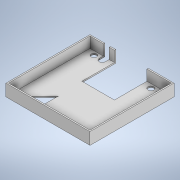
# Autodesk Inventor part: FixedLid
Saved by Autodesk Inventor 2020 (Build 240168000, 168)
## iProperties
Created: 2020-04-03
Part Number: FixedLid
Material: Generic
Document SubType Name: Modeling
Designer: jared.jones280
Density: 1 g/cm^3
Appearance: Default
Author: jared.jones280
Autodesk Inventor part; units mm, degrees
ref_plane "YZ Plane" through (0, 0, 0) normal (1, 0, 0) x (0, 1, 0)
ref_plane "XZ Plane" through (0, 0, 0) normal (0, 1, 0) x (-1, 0, 0)
ref_plane "XY Plane" through (0, 0, 0) normal (0, 0, 1) x (1, 0, 0)
sketch "Sketch1" plane through (0, 0, 0) normal (0, 1, 0) x (-1, 0, 0)
  line L0 (0, 0) -> (-195, 0)
  line L1 (-195, 0) -> (-195, -195)
  line L2 (-195, -195) -> (0, -195)
  line L3 (0, -195) -> (0, 0)
  line L4 (3.175, 3.175) -> (-198.1708, 3.175)
  line L5 (-198.1708, 3.175) -> (-198.1708, -198.1708)
  line L6 (-198.1708, -198.1708) -> (3.175, -198.1708)
  line L7 (3.175, -198.1708) -> (3.175, 3.175)
  dimension "d0" = 195
  dimension "d1" = 195
  dimension "d2" = 201.3458
  dimension "d3" = 201.3458
  constraints: 16 end point, 4 parallel, 2 horizontal, 2 perpendicular
  measures "d0" distance of L2.end L1.end
  measures "d1" distance of L1.end L0.end
  measures "d2" distance of L6.end L5.end
  measures "d3" distance of L5.end L4.end
extrude "Extrusion1" add sketch "Sketch1" along normal blind 25.4
sketch "Sketch2" plane through (0, 0, 0) normal (0, 1, 0) x (-1, 0, 0)
  line L0 (3.175, 3.175) -> (-198.1708, 3.175) projected
  line L1 (3.175, -198.1708) -> (3.175, 3.175) projected
  line L2 (-198.1708, 3.175) -> (-198.1708, -198.1708) projected
  line L3 (-198.1708, -198.1708) -> (3.175, -198.1708) projected
  point P0 (0, 0)
extrude "Extrusion2" add sketch "Sketch2" against normal blind 3.175
sketch "Sketch3" plane through (0, 0, 0) normal (0, 1, 0) x (1, 0, 0)
  line L0 (0, 195) -> (195, 195) projected
  line L1 (0, 195) -> (97.4979, 195)
  line L2 (97.4979, 195) -> (136.4979, 195)
  line L3 (97.4979, 195) -> (136.4979, 195) construction
  line L4 (136.4979, 195) -> (58.5199, 195)
  line L5 (58.5199, 195) -> (58.5199, 117.022)
  line L6 (58.5199, 117.022) -> (136.4979, 117.022)
  line L7 (136.4979, 117.022) -> (136.4979, 195)
  point P0 (0, 0)
  dimension "d8" = 97.4979
  dimension "d9" = 39
  dimension "d10" = 0
  dimension "d11" = 77.978
  dimension "d12" = 77.978
  constraints: 14 end point, 2 collinear, 2 horizontal, 2 parallel, 1 perpendicular, 1 point on line
  measures "d8" distance of L0.start L1.end
  measures "d9" distance of L1.end L2.end
  measures "d10" distance between parallel lines of L2 L3
  measures "d11" distance of L6.end L5.end
  measures "d12" distance of L5.end L4.end
extrude "Extrusion3" cut sketch "Sketch3" against normal blind 3.175
sketch "Sketch4" plane through (0, 0, 0) normal (0, 1, 0) x (1, 0, 0)
  line L0 (0, 0) -> (0, 195) projected
  line L1 (0, 195) -> (195, 195) projected
  line L2 (58.5199, 117.022) -> (58.5199, 195) projected
  line L3 (136.4979, 195) -> (136.4979, 117.022) projected
  line L4 (195, 195) -> (195, 0) projected
  line L5 (0, 0) -> (0, 195) projected
  line L6 (0, 195) -> (19.5072, 195)
  line L7 (19.5072, 195) -> (39.0144, 195)
  line L8 (0, 195) -> (0, 185)
  circle A0 centre (19.5072, 185) radius 6.5
  circle A1 centre (39.0144, 185) radius 7
  line L9 (136.4979, 195) -> (195, 195) projected
  line L10 (195, 195) -> (195, 184.9924)
  line L11 (198.1708, 198.1708) -> (198.1708, -3.175) projected
  line L12 (195, 195) -> (205.0076, 195) construction
  line L13 (195, 195) -> (175.4928, 195)
  line L14 (195, 195) -> (214.5072, 195) construction
  line L15 (175.4928, 195) -> (155.9856, 195)
  circle A2 centre (175.4928, 184.9924) radius 6.5024
  circle A3 centre (155.9856, 184.9924) radius 6.9977
  dimension "d15" = 58.5199
  dimension "d16" = 19.5072
  dimension "d17" = 19.5072
  dimension "d18" = 10
  dimension "d19" = 13
  dimension "d20" = 14
  dimension "d21" = 10.0076
  dimension "d22" = 90
  dimension "d23" = 19.5072
  dimension "d24" = 180
  dimension "d25" = 19.5072
  dimension "d26" = 13.0048
  dimension "d27" = 13.9954
  constraints: 16 end point, 4 centre point, 4 point on line, 2 equal length, 2 horizontal, 1 collinear, 1 parallel
  measures "d15" distance from line of L0 L2.end
  measures "d16" distance of L0.end L6.end
  measures "d17" distance of L6.end L7.end
  measures "d18" distance of L0.end L8.end
  measures "d19" diameter of A0
  measures "d20" diameter of A1
  measures "d21" distance of L1.end L10.end
  measures "d22" angle of L10 L12
  measures "d23" distance of L1.end L13.end
  measures "d24" angle of L13 L14
  measures "d25" distance of L13.end L15.end
  measures "d26" diameter of A2
  measures "d27" diameter of A3
extrude "Extrusion4" cut sketch "Sketch4" against normal blind 3.175
sketch "Sketch5" plane through (0, -3.175, 0) normal (0, -1, 0) x (1, 0, 0)
  circle A0 centre (61.0901, -58.3837) radius 57.15
  line L0 (61.0901, -58.3837) -> (61.0901, -1.2337)
  line L1 (61.0901, -58.3837) -> (118.2401, -58.3837) construction
  line L2 (61.0901, -58.3837) -> (20.679, -17.9725)
  line L3 (61.0901, -58.3837) -> (118.2401, -58.3837) construction
  point P0 (0, 0)
  dimension "d32" = 114.3
  dimension "d33" = 57.15
  dimension "d34" = 90
  dimension "d35" = 57.15
  dimension "d36" = 135
  constraints: 8 end point, 2 equal length, 2 horizontal, 1 centre point, 1 vertical
  measures "d32" diameter of A0
  measures "d33" distance of L0.start L0.end
  measures "d34" angle of L1 L0
  measures "d35" distance of L0.start L2.end
  measures "d36" angle of L3 L2
extrude "Extrusion5" cut sketch "Sketch5" against normal blind 3.175 contours L0 L2 A0 picked at (52.2233, -21.4506)
sketch "Sketch6" plane through (0, -3.175, 0) normal (0, -1, 0) x (1, 0, 0)
  line L0 (136.4979, -195) -> (58.5199, -195) projected
  line L1 (-3.175, -198.1708) -> (198.1708, -198.1708) projected
  line L2 (136.4979, -195) -> (58.5199, -195)
  line L3 (58.5199, -195) -> (58.5199, -198.175)
  line L4 (58.5199, -198.175) -> (136.4979, -198.175)
  line L5 (136.4979, -198.175) -> (136.4979, -195)
  point P0 (0, 0)
  point P1 (136.4979, -198.1708)
  point P2 (58.5199, -198.1708)
  dimension "d39" = 3.175
  constraints: 8 end point, 2 parallel, 1 horizontal, 1 perpendicular
  measures "d39" distance of L3.end L2.end
extrude "Extrusion6" cut sketch "Sketch6" against normal through all contours L5 L1 L3 L0
sketch "Sketch7" plane through (0, -3.175, 0) normal (0, -1, 0) x (1, 0, 0)
  circle A0 centre (39.0144, -185) radius 7 projected
  line L0 (58.5199, -198.1708) -> (-3.175, -198.1708) projected
  line L1 (32.0144, -185) -> (46.0098, -185)
  line L2 (46.0098, -185) -> (46.0098, -198.1708)
  line L3 (46.0098, -198.1708) -> (32.0144, -198.1708)
  line L4 (32.0144, -198.1708) -> (32.0144, -185)
  point P0 (0, 0)
  dimension "d42" = 13.9954
  constraints: 8 end point, 2 parallel, 1 horizontal, 1 horizontal alignment, 1 perpendicular, 1 point on line, 1 other
  measures "d42" distance of L2.end L3.end
extrude "Extrusion7" cut sketch "Sketch7" against normal through all contours L1 L2 A0 | A0 L2 L0 L4 picked at (36.7458, -185.5521)
body "Solid1"
